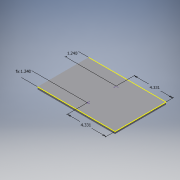
# Autodesk Inventor part: BS #2
Saved by Autodesk Inventor 2019 (Build 230136000, 136)
## iProperties
Created: 2019-02-18
Part Number: BS #2
Material: Generic
Document SubType Name: Modeling
Designer: Tesler
Density: 1 g/cm^3
Appearance: Default
Author: Tesler
Autodesk Inventor part; units mm, degrees
ref_plane "YZ Plane" through (0, 0, 0) normal (1, 0, 0) x (0, 1, 0)
ref_plane "XZ Plane" through (0, 0, 0) normal (0, 1, 0) x (-1, 0, 0)
ref_plane "XY Plane" through (0, 0, 0) normal (0, 0, 1) x (1, 0, 0)
sketch "Sketch1" plane through (0, 0, 0) normal (0, 1, 0) x (-1, 0, 0)
  line L0 (0, 0) -> (220.0001, 0)
  line L1 (220.0001, 0) -> (220.0001, -145)
  line L2 (220.0001, -145) -> (0, -145)
  line L3 (0, -145) -> (0, 0)
  dimension "d0" = 220.0001
  dimension "d1" = 145
  constraints: 8 end point, 2 parallel, 1 horizontal, 1 perpendicular
  measures "d0" distance of L1.end L2.end
  measures "d1" distance of L0.end L1.end
extrude "Extrusion1" add sketch "Sketch1" along normal blind 6.35
sketch "Sketch4" plane through (0, 6.35, 0) normal (0, 1, 0) x (1, 0, 0)
  line L0 (0, 145) -> (-220.0001, 145) projected
  line L1 (-220.0001, 0) -> (0, 0) projected
  line L2 (0, 0) -> (0, 145) projected
  point P0 (-110, 113.5)
  point P1 (-110, 31.5)
  dimension "d24" = 31.5
  dimension "d25" = 31.5
  dimension "d26" = 110
  dimension "d27" = 110
  measures "d24" distance from line of L0 point (-110, 113.5)
  measures "d25" distance from line of L1 point (-110, 31.5)
  measures "d26" distance from line of L2 point (-110, 113.5)
  measures "d27" distance from line of L2 point (-110, 31.5)
equation "\"d25\" = d24"
body "Solid1"
